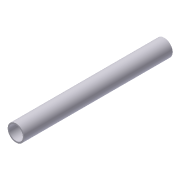
# Autodesk Inventor part: FE-00018-01
Saved by Autodesk Inventor 2012 (Build 160160000, 160)
## iProperties
Company: FIRST
Created: 2008-05-30
Part Number: FE-00018-01
Document SubType Name: Modeling
Designer: dfoster
Density: 1 g/cm^3
Description: Connecting Tube
Mass: 161.687 g
Surface Area: 914.771 cm^2
Volume: 161.687 cm^3
Material: Default
Title: Connecting Tube
Author: dfoster
Autodesk Inventor part; units mm, degrees
ref_plane "YZ Plane" through (0, 0, 0) normal (1, 0, 0) x (0, 1, 0)
ref_plane "XZ Plane" through (0, 0, 0) normal (0, 1, 0) x (-1, 0, 0)
ref_plane "XY Plane" through (0, 0, 0) normal (0, 0, 1) x (1, 0, 0)
sketch "Sketch1" plane through (0, 0, 0) normal (0, 0, 1) x (1, 0, 0)
  circle A0 centre (0, 0) radius 21.0312
  circle A1 centre (0, 0) radius 17.4625
  dimension "d0" = 42.0624
  dimension "d1" = 34.925
  constraints: 2 centre point, 1 coincident
  measures "d0" diameter of A0
  measures "d1" diameter of A1
extrude "Extrusion1" add sketch "Sketch1" along normal blind 374.65
body "Solid1"
